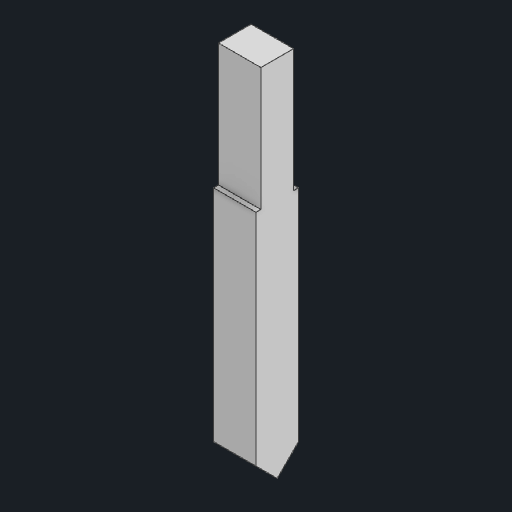
# Autodesk Inventor part: ForearmActuatorBodyBoundingBoxReal
Saved by Autodesk Inventor 2023 (Build 270158000, 158)
## iProperties
Created: 2023-03-25
Part Number: ForearmActuatorBodyBoundingBoxReal
Material: Generic
Document SubType Name: Modeling
Designer: Val
Density: 1 g/cm^3
Appearance: Default
Author: Val
Autodesk Inventor part; units mm, degrees
ref_plane "YZ Plane" through (0, 0, 0) normal (1, 0, 0) x (0, 1, 0)
ref_plane "XZ Plane" through (0, 0, 0) normal (0, 1, 0) x (-1, 0, 0)
ref_plane "XY Plane" through (0, 0, 0) normal (0, 0, 1) x (1, 0, 0)
sketch "Sketch1" plane through (0, 0, 0) normal (1, 0, 0) x (0, 1, 0)
  line L0 (0, 13) -> (134.5, 13)
  line L1 (134.5, 13) -> (134.5, -13)
  line L2 (134.5, -13) -> (0, -13)
  line L3 (0, -13) -> (0, 13) construction
  line L4 (134.5, 10) -> (209.702, 10)
  line L5 (209.702, 10) -> (209.702, -10)
  line L6 (209.702, -10) -> (134.5, -10)
  line L7 (134.5, -10) -> (134.5, 10)
  line L8 (134.5, 10) -> (208.702, 10) construction
  line L9 (133, 13) -> (0, 13) construction
  line L10 (133, -13) -> (8.0257, -13) construction
  line L11 (0, 13) -> (-13, 0)
  line L12 (-13, 0) -> (0, -13)
  line L13 (-57.5404, 0) -> (254.2424, 0) construction
  arc A0 (0, 13) -> (-8.5144, -9.8237) centre (0, 0) ccw construction
  circle A1 centre (0, 0) radius 11.5 projected
  circle A2 centre (0, 0) radius 9 projected
  point P0 (209.702, 0)
  constraints: 28 end point, 6 horizontal, 4 parallel, 3 collinear, 3 point on circle, 2 perpendicular, 2 point on line, 1 centre point, 1 midpoint, 12 other
extrude "Extrusion1" add sketch "Sketch1" along normal mid plane 26 contours L0 L1 L2 L12 A1 L11 | A1 L12 L11 | L4 L5 L6 L1 | A1 L12 L11 | A2
body "Solid1"
